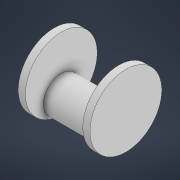
# Autodesk Inventor part: 軸
Saved by Autodesk Inventor 2021 (Build 250183000, 183)
## iProperties
Created: 2020-12-28
Part Number: 軸
Material: 一般
Document SubType Name: Modeling
Designer: zihon
Density: 1 g/cm^3
Appearance: 預設
Author: zihon
Autodesk Inventor part; units mm, degrees
ref_plane "YZ Plane" through (0, 0, 0) normal (1, 0, 0) x (0, 1, 0)
ref_plane "XZ Plane" through (0, 0, 0) normal (0, 1, 0) x (-1, 0, 0)
ref_plane "XY Plane" through (0, 0, 0) normal (0, 0, 1) x (1, 0, 0)
sketch "草圖1" plane through (0, 0, 0) normal (1, 0, 0) x (0, 1, 0)
  circle A0 centre (0, 0) radius 0.25
  arc A1 (0, 0.25) -> (0, -0.25) centre (0, 0) ccw
  circle A2 centre (0.25, 0) radius 0.5
  line L0 (-0.45, 0) -> (0.95, 0) projected
  point P0 (-0.25, 0)
  dimension "d44" = 0.5
  dimension "d49" = 1
  constraints: 3 centre point, 2 point on circle, 1 coincident, 1 midpoint, 1 tangent
  measures "d44" diameter of A0
  measures "d49" diameter of A2
extrude "擠出11" add sketch "草圖1" along normal mid plane 1
extrude "擠出12" cut sketch "草圖1" along normal mid plane 0.8 contours L0 A2 A0 | A0 A2 L0
